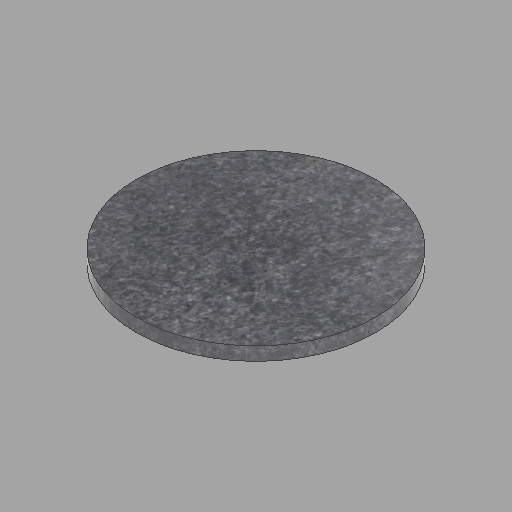
# Autodesk Inventor part: 2x36x36-1
Saved by Autodesk Inventor 2023 (Build 270158000, 158)
## iProperties
Created: 2022-02-10
Part Number: 2x36x36-1
Material: Granite, Cut, Polished
Document SubType Name: Modeling
Designer: awelt
Mass: 90072 g
Surface Area: 14593.2 cm^2
Volume: 33360 cm^3
Density: 2.7 g/cm^3
Appearance: Kasota SN sapphire
TEST: 0.001
Author: awelt
Autodesk Inventor part; units mm, degrees
ref_plane "YZ Plane" through (0, 0, 0) normal (1, 0, 0) x (0, 1, 0)
ref_plane "XZ Plane" through (0, 0, 0) normal (0, 1, 0) x (-1, 0, 0)
ref_plane "XY Plane" through (0, 0, 0) normal (0, 0, 1) x (1, 0, 0)
sketch "Sketch1" plane through (0, 0, 0) normal (1, 0, 0) x (0, 1, 0)
  line L0 (0, 0) -> (50.8, 0)
  line L1 (50.8, 0) -> (50.8, 914.4)
  line L2 (50.8, 914.4) -> (0, 914.4)
  line L3 (0, 914.4) -> (0, 0)
  dimension "d0" = 50.8
  dimension "d1" = 914.4
  constraints: 8 end point, 2 parallel, 1 horizontal, 1 perpendicular
  measures "d0" distance of L2.end L1.end
  measures "d1" distance of L1.end L0.end
extrude "Extrusion1" add sketch "Sketch1" along normal blind 914.4
sketch "Sketch2" plane through (0, 50.8, 914.4) normal (0, 1, 0) x (1, 0, 0)
  line L0 (0, 914.4) -> (0, 0) projected
  line L1 (0, 0) -> (914.4, 0) projected
  line L2 (914.4, 914.4) -> (914.4, 0) projected
  line L3 (0, 914.4) -> (914.4, 914.4) projected
  line L4 (0, 914.4) -> (914.4, 914.4) construction
  line L5 (457.2, 914.4) -> (457.2, 0) construction
  circle A0 centre (457.2, 457.2) radius 457.2
  point P0 (0, 457.2)
  point P1 (914.4, 457.2)
  point P2 (457.2, 0)
  constraints: 3 midpoint, 2 end point, 1 centre point
extrude "Extrusion2" cut sketch "Sketch2" along normal through all both and the other way through all contours L3 A0 L0 | A0 L1 L0 | L3 L2 A0 | A0 L2 L1
body "Solid1"
